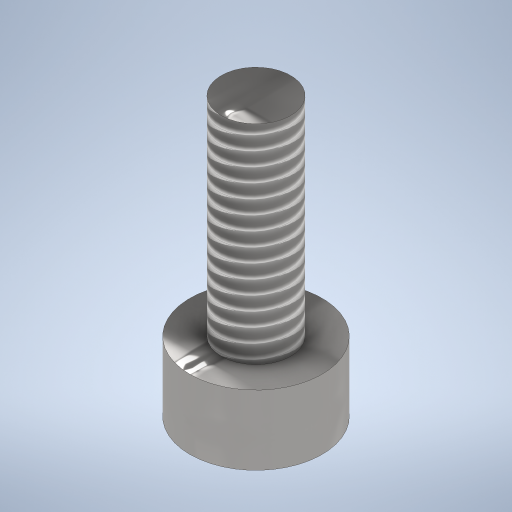
# Autodesk Inventor part: UC-0206
Saved by Autodesk Inventor 2024.2 (Build 282272000, 272)
## iProperties
Created: 2024-01-03
Part Number: UC-0206
Material: Stainless Steel AISI 304
Document SubType Name: Modeling
Designer: Masato Kubotera
Density: 8 g/cm^3
Appearance: Satin Hammered
Vendor: NISSAN SCREW
Catalog Web Link: https://wilco.jp/products/U/UC.html#page1
Mass: 0.417197 g
Surface Area: 1.14586 cm^2
Volume: 0.0521497 cm^3
Author: Masato Kubotera
Autodesk Inventor part; units mm, degrees
ref_plane "YZ Plane" through (0, 0, 0) normal (1, 0, 0) x (0, 1, 0)
ref_plane "XZ Plane" through (0, 0, 0) normal (0, 1, 0) x (-1, 0, 0)
ref_plane "XY Plane" through (0, 0, 0) normal (0, 0, 1) x (1, 0, 0)
sketch "Sketch1" plane through (0, 0, 0) normal (0, 1, 0) x (-1, 0, 0)
  line L0 (0, 0) -> (-1.9, 0)
  line L1 (-1.9, 0) -> (-1.9, 2)
  line L2 (-1.9, 2) -> (-1, 2)
  line L3 (-1, 2) -> (-1, 8)
  line L4 (-1, 8) -> (0, 8)
  line L5 (0, 8) -> (0, 0)
  dimension "ScrewLength" = 6
  dimension "Diameter" = 3.8
  dimension "Metric" = 2
  dimension "HeadLength" = 2
  constraints: 12 end point, 3 horizontal, 3 vertical
  measures "ScrewLength" distance of L2.end L3.end
  measures "Diameter" diameter of L1 L5
  measures "Metric" diameter of L3 L5
  measures "HeadLength" distance of L0.end L1.end
revolve "Revolution1" add sketch "Sketch1" angle 360 about axis through (0, 0, 8) along (0, 0, -1)
thread "Thread1" size "M2x0.4" class "6g" standard "ANSI Metric M Profile" full length
sketch "Sketch2" plane through (0, 0, 0) normal (0, 0, -1) x (-1, 0, 0)
  line L0 (0.433, 0.75) -> (0.866, 0)
  line L1 (0.866, 0) -> (0.433, -0.75)
  line L2 (0.433, -0.75) -> (-0.433, -0.75)
  line L3 (-0.433, -0.75) -> (-0.866, 0)
  line L4 (-0.866, 0) -> (-0.433, 0.75)
  line L5 (-0.433, 0.75) -> (0.433, 0.75)
  point P0 (0, 0)
  point P1 (0, 0)
  dimension "WidthAcrossFlat" = 1.5
  constraints: 12 end point, 1 coincident, 1 horizontal, 13 other
  measures "WidthAcrossFlat" distance between parallel lines of L2 L5
extrude "Extrusion1" cut sketch "Sketch2" against normal blind 1
body "Solid1"
